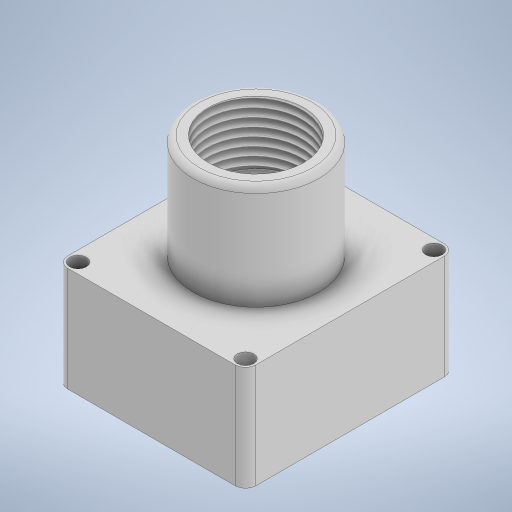
# Autodesk Inventor part: Practica No. 1 Oscar Bustamante
Saved by Autodesk Inventor 2024 (Build 280153000, 153)
## iProperties
Created: 2024-02-19
Part Number: Practica No. 1 Oscar Bustamante
Material: Genérico
Document SubType Name: Modeling
Designer: Admin
Density: 1 g/cm^3
Appearance: Valor por defecto
Author: Admin
Autodesk Inventor part; units mm, degrees
ref_plane "YZ Plane" through (0, 0, 0) normal (1, 0, 0) x (0, 1, 0)
ref_plane "XZ Plane" through (0, 0, 0) normal (0, 1, 0) x (-1, 0, 0)
ref_plane "XY Plane" through (0, 0, 0) normal (0, 0, 1) x (1, 0, 0)
sketch "Boceto1" plane through (0, 0, 0) normal (0, 1, 0) x (-1, 0, 0)
  point P0 (0, 0)
sketch "Boceto2" plane through (0, 0, 0) normal (0, 1, 0) x (-1, 0, 0)
  line L0 (-45, -50) -> (45, -50)
  line L1 (45, -50) -> (45, 50)
  line L2 (45, 50) -> (-45, 50)
  line L3 (-45, 50) -> (-45, -50)
  line L4 (-45, -50) -> (45, 50) construction
  line L5 (45, -50) -> (-45, 50) construction
  point P0 (0, 0)
  dimension "d0" = 90
  dimension "d1" = 100
  constraints: 12 end point, 2 midpoint, 2 parallel, 1 horizontal, 1 perpendicular
  measures "d0" distance of L2.end L1.end
  measures "d1" distance of L1.end L0.end
extrude "Extrusión1" add sketch "Boceto2" along normal blind 50
sketch "Boceto3" plane through (0, 50, 0) normal (0, 1, 0) x (1, 0, 0)
  point P0 (0, 0)
  point P1 (0, 0)
  constraints: 1 coincident
sketch "Boceto4" plane through (0, 50, 0) normal (0, 1, 0) x (1, 0, 0)
  circle A0 centre (0, 0) radius 30
  dimension "d4" = 60
  constraints: 1 centre point, 1 coincident
  measures "d4" diameter of A0
extrude "Extrusión2" add sketch "Boceto4" along normal blind 50
sketch "Boceto5" plane through (0, 100, 0) normal (0, 1, 0) x (1, 0, 0)
  point P0 (0, 0)
  point P1 (0, 0)
  constraints: 1 coincident
fillet "Empalme1" radius 3 1 edges at (-30, 100, 0)
hole "Agujero1" at (0, 100, 0) direction (0, -1, 0) diameter 45.6699 depth 30 thread size "M50x4" class "6H" standard "ANSI Metric M Profile"
fillet "Empalme2" radius 5 1 edges at (45, 25, 50)
fillet "Empalme3" radius 5 1 edges at (-45, 25, 50)
fillet "Empalme4" radius 5 1 edges at (45, 25, -50)
fillet "Empalme5" radius 5 1 edges at (-45, 25, -50)
sketch "Boceto9" plane through (0, 50, 0) normal (0, 1, 0) x (1, 0, 0)
  arc A0 (-40, 50) -> (-45, 45) centre (-40, 45) ccw projected
  circle A1 centre (-40, 45) radius 4
  arc A2 (45, 45) -> (40, 50) centre (40, 45) ccw projected
  circle A3 centre (40, 45) radius 4
  arc A4 (-45, -45) -> (-40, -50) centre (-40, -45) ccw projected
  circle A5 centre (-40, -45) radius 4
  arc A6 (40, -50) -> (45, -45) centre (40, -45) ccw projected
  circle A7 centre (40, -45) radius 4
  point P0 (0, 0)
  dimension "d28" = 8
  dimension "d29" = 8
  dimension "d30" = 8
  dimension "d31" = 8
  constraints: 4 centre point, 4 coincident
  measures "d28" diameter of A1
  measures "d29" diameter of A3
  measures "d30" diameter of A5
  measures "d31" diameter of A7
hole "Agujero2" at (-40, 50, 45) at (-40, 50, -45) at (40, 50, -45) at (40, 50, 45) direction (0, -1, 0) diameter 8 depth 50
